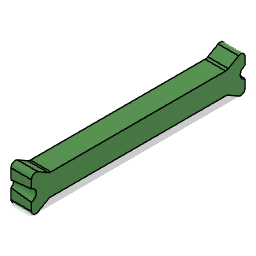
strut (Autodesk Fusion 360 design; units mm, degrees)
Autodesk Fusion 360 part; units mm, degrees
sketch "Sketch1" plane through (0, 0, 0) normal (1, 0, 0) x (0, 0, -1)
  arc A0 (5.5, 0) -> (0.9551, 5.4164) centre (0, 0) ccw
  line L0 (0.9551, 5.4164) -> (0, 0) construction
  line L1 (5.5, 0) -> (0, 0) construction
  line L2 (6.9551, 16.1918) -> (16.5192, 10.6699)
  arc A1 (16.5192, 10.6699) -> (19.0192, 10) centre (19.0192, 15) ccw
  line L3 (19.0192, 10) -> (100, 10)
  arc A2 (6.9551, 16.1918) -> (0.9551, 12.7276) centre (4.9551, 12.7276) ccw
  line L4 (100, 10) -> (100, 0)
  line L5 (0.9551, 12.7276) -> (0.9551, 5.4164)
  line L6 (2.75, 4.7631) -> (9.0817, 1.1075) construction
  line L7 (0.9551, 5.4164) -> (0.9551, 0)
  line L8 (0.9551, 0) -> (100, 0)
  circle A3 centre (0, 0) radius 5.5
  dimension "d7" = 80
  dimension "d8" = 30
  dimension "d10" = 4
  dimension "d14" = 10
  dimension "d16" = 5
  dimension "d17" = 100
  dimension "d18" = 5.5
  dimension "d21" = 12
  constraint coincident A0.centre L0.end
  constraint horizontal L1
  constraint tangent L2 A1
  constraint tangent A1 L3
  constraint parallel L1 L3
  constraint tangent L2 A2
  constraint perpendicular L3 L4
  constraint coincident L1 L4.end
  constraint perpendicular L1 L5
  constraint tangent A2 L5
  constraint coincident A0 L6.start
  constraint tangent A0 L6
  constraint equal L5 L6
  constraint parallel L2 L6
  constraint coincident L1 L7.end
  constraint perpendicular L1 L7
  constraint coincident A0.end A3
  measures "d7" angle of L0 L1
  measures "d8" angle of L1 L2
  measures "d10" radius of A2
  measures "d14" distance of L1 L3
  measures "d16" radius of A1
  measures "d17" distance of A0.centre L4
  measures "d18" radius of A0
  measures "d21" distance of L2 L6
extrude "Extrude1" add sketch "Sketch1" against normal blind 19 contours A0 L7 L8 A3 | A0 L2 A1 L3 A2 L4 L5 L8 A3
extrude "Extrude2" cut sketch "Sketch1" against normal up to surface (19 mm away) draft -6.6 contours A0 L7 L8 A3 | L7 L8 A3
mirror "Mirror1" about plane through (0, 0, -5.5) normal (0, -1, 0) of bodies 1 merged
mirror "Mirror2" about plane through (0, 10, -100) normal (0, 0, -1) of bodies 1 merged
sketch "Sketch2" plane through (0, 0, 0) normal (1, 0, 0) x (0, 0, -1)
  arc A0 (0.9551, -5.4164) -> (0.9551, 5.4164) centre (0, 0) ccw
  line L0 (0.9551, -5.4164) -> (0.9551, -12.7276)
  arc A1 (0.9551, -12.7276) -> (6.9551, -16.1918) centre (4.9551, -12.7276) ccw
  line L1 (6.9551, -16.1918) -> (16.5192, -10.6699)
  arc A2 (19.0192, -10) -> (16.5192, -10.6699) centre (19.0192, -15) ccw
  line L2 (19.0192, -10) -> (180.9808, -10)
  arc A3 (183.4808, -10.6699) -> (180.9808, -10) centre (180.9808, -15) ccw
  line L3 (183.4808, -10.6699) -> (193.0449, -16.1918)
  arc A4 (193.0449, -16.1918) -> (199.0449, -12.7276) centre (195.0449, -12.7276) ccw
  line L4 (199.0449, -12.7276) -> (199.0449, -5.4164)
  arc A5 (199.0449, 5.4164) -> (199.0449, -5.4164) centre (200, 0) ccw
  line L5 (199.0449, 5.4164) -> (199.0449, 12.7276)
  arc A6 (199.0449, 12.7276) -> (193.0449, 16.1918) centre (195.0449, 12.7276) ccw
  line L6 (193.0449, 16.1918) -> (183.4808, 10.6699)
  arc A7 (180.9808, 10) -> (183.4808, 10.6699) centre (180.9808, 15) ccw
  line L7 (180.9808, 10) -> (19.0192, 10)
  arc A8 (16.5192, 10.6699) -> (19.0192, 10) centre (19.0192, 15) ccw
  line L8 (16.5192, 10.6699) -> (6.9551, 16.1918)
  arc A9 (6.9551, 16.1918) -> (0.9551, 12.7276) centre (4.9551, 12.7276) ccw
  line L9 (0.9551, 12.7276) -> (0.9551, 5.4164)
  line L10 (16.5192, 25) -> (200, 25)
  line L11 (200, 25) -> (200, -25)
  line L12 (200, -25) -> (16.5192, -25)
  line L13 (16.5192, -25) -> (16.5192, 25)
  dimension "d1" = 25
  dimension "d2" = 25
  constraint horizontal L10
  constraint vertical L11
  constraint horizontal L12
  constraint vertical L13
  constraint coincident A5.centre L11
  constraint coincident A8.start L13
  measures "d1" distance of A5.centre L10
  measures "d2" distance of A5.centre L12
extrude "Extrude3" [suppressed]
